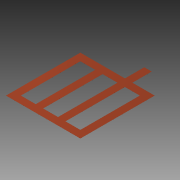
# Autodesk Inventor part: Square_Copper
Saved by Autodesk Inventor 2014 SP1 (Build 180222100, 222)
## iProperties
Created: 2014-01-12
Part Number: Square_Copper
Material: Copper
Document SubType Name: Modeling
Designer: tuleu
Density: 8.94 g/cm^3
Appearance: Copper - Satin
Author: tuleu
Autodesk Inventor part; units mm, degrees
ref_plane "YZ Plane" through (0, 0, 0) normal (1, 0, 0) x (0, 1, 0)
ref_plane "XZ Plane" through (0, 0, 0) normal (0, 1, 0) x (-1, 0, 0)
ref_plane "XY Plane" through (0, 0, 0) normal (0, 0, 1) x (1, 0, 0)
sketch "Sketch1" plane through (0, 0, 0) normal (0, 0, 1) x (1, 0, 0)
  line L0 (62.5, -62.5) -> (-62.5, -62.5)
  line L1 (50, -50) -> (50, 50)
  line L2 (50, 62.5) -> (62.5, 62.5)
  line L3 (62.5, 62.5) -> (62.5, -62.5)
  line L4 (75, -75) -> (-75, -75) construction
  line L5 (-75, -75) -> (-75, 75) construction
  line L6 (-75, 75) -> (75, 75) construction
  line L7 (75, 75) -> (75, -75) construction
  line L8 (0, -75) -> (0, 75) construction
  line L9 (75, 0) -> (-75, 0) construction
  line L10 (12.5, -50) -> (12.5, 50)
  line L11 (25, 50) -> (25, -50)
  line L12 (-25, -50) -> (-25, 50)
  line L13 (-12.5, 50) -> (-12.5, -50)
  line L14 (-62.5, -62.5) -> (-62.5, 62.5)
  line L15 (-50, 50) -> (-50, -50)
  line L16 (-62.5, -62.5) -> (-62.5, -50)
  line L17 (62.5, -50) -> (62.5, -62.5)
  line L18 (-62.5, 62.5) -> (-62.5, 50)
  line L19 (62.5, 50) -> (62.5, 62.5)
  line L20 (25, -50) -> (50, -50)
  line L21 (-50, -50) -> (-25, -50)
  line L22 (-12.5, -50) -> (12.5, -50)
  line L23 (25, 50) -> (50, 50)
  line L24 (-50, 50) -> (-25, 50)
  line L25 (-12.5, 50) -> (12.5, 50)
  line L26 (12.5, 62.5) -> (12.5, 95)
  line L27 (12.5, 95) -> (25, 95)
  line L28 (25, 95) -> (25, 62.5)
  line L29 (62.5, 62.5) -> (25, 62.5)
  line L30 (12.5, 62.5) -> (-62.5, 62.5)
  point P0 (0, 0)
  dimension "d1" = 125
  dimension "d2" = 150
  dimension "d3" = 25
  dimension "d4" = 25
  dimension "d5" = 25
  dimension "d8" = 12.5
  dimension "d9" = 12.5
  dimension "d10" = 12.5
  dimension "d11" = 12.5
  dimension "d13" = 12.5
  dimension "d14" = 12.5
  dimension "d15" = 20
  constraints: 62 end point, 16 parallel, 7 collinear, 6 midpoint, 5 perpendicular, 4 horizontal, 2 point on line, 2 other
  measures "d1" distance of L2.end L0.start
  measures "d2" distance of L4.start L4.end
  measures "d3" distance between parallel lines of L11 L1
  measures "d4" distance between parallel lines of L13 L10
  measures "d5" distance between parallel lines of L15 L12
  measures "d8" distance between parallel lines of L3 L1
  measures "d9" distance between parallel lines of L10 L11
  measures "d10" distance between parallel lines of L12 L13
  measures "d11" distance between parallel lines of L14 L15
  measures "d13" distance between parallel lines of L0 L20
  measures "d14" distance between parallel lines of L29 L23
  measures "d15" distance between parallel lines of L27 L6
extrude "Extrusion1" add sketch "Sketch1" along normal blind 0.01
body "Solid1"
